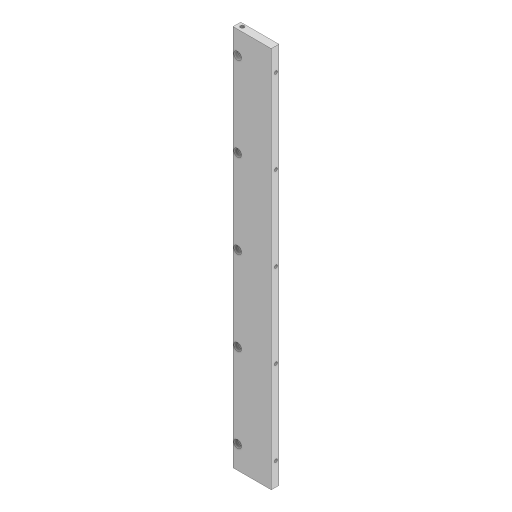
# Autodesk Inventor part: Platte-2
Saved by Autodesk Inventor 2024.3 (Build 283343000, 343)
## iProperties
Created: 2025-05-16
Part Number: Platte-2
Material: Generisch
Document SubType Name: Modeling
Designer: Demir
Density: 1 g/cm^3
Appearance: Vorgabe
Author: Demir
Autodesk Inventor part; units mm, degrees
ref_plane "YZ Plane" through (0, 0, 0) normal (1, 0, 0) x (0, 1, 0)
ref_plane "XZ Plane" through (0, 0, 0) normal (0, 1, 0) x (-1, 0, 0)
ref_plane "XY Plane" through (0, 0, 0) normal (0, 0, 1) x (1, 0, 0)
sketch "Skizze1" plane through (0, 0, 0) normal (0, 0, 1) x (1, 0, 0)
  line L0 (-25, 5) -> (25, 5)
  line L1 (25, 5) -> (25, -5)
  line L2 (25, -5) -> (-25, -5)
  line L3 (-25, -5) -> (-25, 5)
  line L4 (-25, 5) -> (25, -5) construction
  line L5 (25, 5) -> (-25, -5) construction
  point P0 (0, 0)
  dimension "d0" = 50
  dimension "d1" = 10
  constraints: 12 end point, 2 midpoint, 2 parallel, 1 horizontal, 1 perpendicular
  measures "d0" distance of L0.start L0.end
  measures "d1" distance of L2.end L0.start
extrude "Extrusion1" add sketch "Skizze1" along normal mid plane 500
sketch "Skizze4" plane through (-25, -5, 250) normal (0, -1, 0) x (1, 0, 0)
  line L0 (50, -500) -> (50, 0) projected
  line L1 (0, 0) -> (50, 0) projected
  line L2 (0, 0) -> (0, -500) projected
  line L3 (50, -500) -> (0, -500) projected
  point P0 (25, -250)
  point P1 (30, -465)
  dimension "d13" = 30
  dimension "d14" = 35
  measures "d13" distance from line of point (30, -465) L2
  measures "d14" distance from line of point (30, -465) L3
hole "Bohrung2" [suppressed]
sketch "Skizze5" plane through (-25, -5, 250) normal (0, -1, 0) x (1, 0, 0)
  line L0 (50, -500) -> (50, 0) projected
  line L1 (0, 0) -> (50, 0) projected
  line L2 (0, 0) -> (0, -500) projected
  line L3 (50, -500) -> (0, -500) projected
  point P0 (25, -250)
  point P1 (6, -250)
  point P2 (0, -250)
  dimension "d22" = 6
  constraints: 1 horizontal alignment, 1 midpoint
  measures "d22" distance of point (6, -250) point (0, -250)
hole "Bohrung3" at (-19, -5, 0) direction (0, 1, 0) diameter 5.5 depth 32.3 tip angle 118 counterbore diameter 10 counterbore depth 5
pattern_linear "Rechteckige Anordnung1" count 3 spacing 110 along (0, 0, -1) count 3 spacing 110 along (0, 0, 1) of "Bohrung3"
sketch "Skizze6" plane through (25, 5, 250) normal (1, 0, 0) x (0, 0, -1)
  line L0 (500, 0) -> (0, 0) projected
  line L1 (0, -10) -> (0, 0) projected
  line L2 (500, -10) -> (0, -10) projected
  line L3 (500, 0) -> (500, -10) projected
  point P0 (250, -5)
  point P1 (250, -4)
  dimension "d60" = 6
  constraints: 1 vertical alignment
  measures "d60" distance from line of point (250, -4) L2
hole "Bohrung4" at (25, 1, 0) direction (-1, 0, 0) diameter 4.134 depth 14.2 tip angle 118 thread size "M5x0.8" class "6H" standard "ISO Metric profile"
pattern_linear "Rechteckige Anordnung2" count 3 spacing 110 along (0, 0, 1) count 3 spacing 110 along (0, 0, -1) of "Bohrung4"
sketch "Skizze7" plane through (0, 0, 250) normal (0, 0, 1) x (1, 0, 0)
  line L0 (-21.75, 5) -> (-21.75, 0) projected
  line L1 (-25, 5) -> (-25, -5) projected
  line L2 (25, 5) -> (-25, 5) projected
  point P0 (0, 0)
  point P1 (-19, 1)
  dimension "d49" = 6
  dimension "d61" = 4
  measures "d49" distance from line of point (-19, 1) L1
  measures "d61" distance from line of point (-19, 1) L2
hole "Bohrung5" at (-19, 1, 250) direction (0, 0, -1) diameter 4.134 depth 14.2 tip angle 118 thread size "M5x0.8" class "6H" standard "ISO Metric profile"
chamfer "Fasen1" distance 0.5 angle 45 1 edges at (-19, 3.067, 250)
